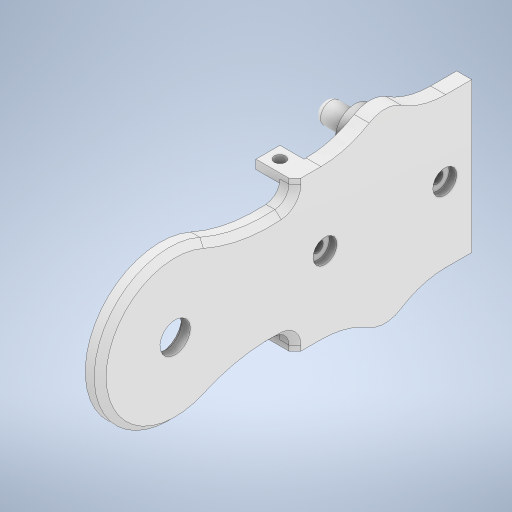
# Autodesk Inventor part: bldc_arm
Saved by Autodesk Inventor 2024.2 (Build 282272000, 272)
## iProperties
Created: 2024-03-15
Part Number: bldc_arm
Material: ABS Plastic
Document SubType Name: Modeling
Designer: jerem
Density: 1.06 g/cm^3
Appearance: Smooth - White
Mass: 32.0643 g
Surface Area: 145.548 cm^2
Volume: 30.2494 cm^3
Author: jerem
Autodesk Inventor part; units mm, degrees
ref_plane "YZ Plane" through (0, 0, 0) normal (1, 0, 0) x (0, 1, 0)
ref_plane "XZ Plane" through (0, 0, 0) normal (0, 1, 0) x (-1, 0, 0)
ref_plane "XY Plane" through (0, 0, 0) normal (0, 0, 1) x (1, 0, 0)
sketch "Sketch1" plane through (0, 0, 0) normal (1, 0, 0) x (0, 1, 0)
  line L0 (0, 0) -> (0, -10) construction
  line L1 (0, -10) -> (0, -50) construction
  circle A0 centre (0, -10) radius 1.905
  circle A1 centre (0, -50) radius 1.905
  line L2 (10, 0) -> (10, -59)
  line L3 (10, -59) -> (0, -59)
  line L4 (0, -59) -> (-10, -59)
  line L5 (-10, -59) -> (-10, 0)
  line L6 (0, 0) -> (10, 0)
  line L7 (0, 0) -> (-10, 0)
  line L8 (0, -50) -> (0, -59) construction
  circle A2 centre (0, 40) radius 25
  line L9 (10, 0) -> (10, 10)
  line L10 (10, 10) -> (-10, 10)
  line L11 (-10, 10) -> (-10, 0)
  arc A3 (22.8049, 29.7561) -> (10, -30) centre (155.8333, -30) ccw
  arc A4 (-10, -30) -> (-22.8049, 29.7561) centre (-155.8333, -30) ccw
  line L12 (0, -30) -> (21, -30) construction
  line L13 (0, -30) -> (-21, -30) construction
  circle A5 centre (21, -30) radius 3.5
  circle A6 centre (-21, -30) radius 3.5
  circle A7 centre (21, -30) radius 10
  circle A8 centre (-21, -30) radius 10
  circle A9 centre (21, -30) radius 6.5
  circle A10 centre (-21, -30) radius 6.5
  line L14 (-10, -59) -> (-25, -59)
  line L15 (10, -59) -> (25, -59)
  arc A11 (-28.9586, -23.9452) -> (-22.8049, 29.7561) centre (-71.0556, 8.082) ccw
  arc A12 (22.8049, 29.7561) -> (28.9586, -23.9452) centre (71.0556, 8.082) ccw
  line L16 (0, 0) -> (15, 0)
  line L17 (10, 0) -> (25, 0)
  line L18 (25, -59) -> (25, -50.3)
  arc A13 (29.3932, -35.4364) -> (25, -50.3) centre (52.3408, -50.3) ccw
  line L19 (25, 0) -> (25, -8.7)
  arc A14 (25, -8.7) -> (29.5297, -24.7804) centre (55.8075, -8.7) ccw
  line L20 (-10, 0) -> (-25, 0)
  line L21 (-25, -59) -> (-25, -50.3)
  arc A15 (-25, -50.3) -> (-29.3932, -35.4364) centre (-52.3408, -50.3) ccw
  line L22 (-25, 0) -> (-25, -8.7)
  arc A16 (-29.5297, -24.7804) -> (-25, -8.7) centre (-55.8075, -8.7) ccw
  circle A17 centre (0, -50) radius 4
  circle A18 centre (0, -10) radius 4
  circle A19 centre (0, 40) radius 7.235
  circle A20 centre (0, 40) radius 5.08
  point P0 (-10, -30)
  point P1 (10, -30)
  point P2 (23.8246, -39.5928)
  point P3 (10, -63.336)
  point P4 (-30.2308, -33.8462)
  point P5 (28.9586, -23.9452)
  point P6 (22.8049, 29.7561)
  point P7 (30.2308, -26.1538)
  point P8 (18.7815, 0)
  point P9 (-18.7815, 0)
  point P10 (-13.1191, 0)
  point P11 (-29.3932, -35.4364)
  dimension "d0" = 3.81
  dimension "d1" = 3.81
  dimension "d2" = 40
  dimension "d3" = 10
  dimension "d5" = 9
  dimension "d7" = 10
  dimension "d8" = 10
  dimension "d9" = 50
  dimension "d12" = 30
  dimension "d13" = 10
  dimension "d14" = 20
  dimension "d30" = 21
  dimension "d31" = 7
  dimension "d32" = 7
  dimension "d33" = 20
  dimension "d34" = 20
  dimension "d38" = 3
  dimension "d48" = 15
  dimension "d55" = 15
  dimension "d56" = 8.7
  dimension "d57" = 8.7
  dimension "d58" = 15
  dimension "d134" = 8
  dimension "d135" = 8
  dimension "d138" = 14.47
  dimension "d157" = 10.16
  constraints: 47 end point, 25 point on circle, 21 centre point, 14 symmetric about line, 11 coincident, 8 point on line, 8 tangent, 6 perpendicular, 5 horizontal, 5 vertical, 4 equal length, 1 midpoint, 5 other
  measures "d0" diameter of A0
  measures "d1" diameter of A1
  measures "d2" distance of L0.end L1.end
  measures "d3" distance of L0.start L0.end
  measures "d5" distance of L3.end L1.end
  measures "d7" distance from line of L12.start L5
  measures "d8" distance between parallel lines of L1 L2
  measures "d9" diameter of A2
  measures "d12" distance from line of A2.centre L10
  measures "d13" distance of L2.start L9.end
  measures "d14" vertical distance of L0.end A3.end
  measures "d30" distance of L12.start L12.end
  measures "d31" diameter of A5
  measures "d32" diameter of A6
  measures "d33" diameter of A7
  measures "d34" diameter of A8
  measures "d38" radial gap between concentric circles of A9 A5
  measures "d48" distance of L4.end L14.end
  measures "d55" distance of L2.start L17.end
  measures "d56" distance of L15.end L18.end
  measures "d57" distance of L17.end L19.end
  measures "d58" distance of L2.end L15.end
  measures "d134" diameter of A17
  measures "d135" diameter of A18
  measures "d138" diameter of A19
  measures "d157" diameter of A20
extrude "Extrusion1" add sketch "Sketch1" along normal blind 5 contours L16 A3 L2 | L2 L3 L4 L5 L7 L6 | L6 L7 L11 L10 L9 | L9 L10 L11 L20 A4 A2 A3 L16 | A3 L16 L17 A12 A7 A13 L18 L15 L2 | A3 A12 L17 L16 | L5 A4 L20 | A2 | L5 L14 L21 A15 A8 A11 L20 A4 | L20 A11 A4 | L17 L19 A14 A7 A12 | A11 A8 A16 L22 L20 | A7 | A8 | A5 | A6 | A9 | A10 | A17 | A18 | A19 | A20
fillet "Face Fillet1" radius 5 1 edges at (2.5, -18.7815, 0)
fillet "Face Fillet2" radius 5 1 edges at (2.5, 18.7815, 0)
extrude "Extrusion16" cut sketch "Sketch1" along normal up to surface (5 mm away) contours A20
extrude "Extrusion17" cut sketch "Sketch1" along normal blind 2 from surface at 0 contours A19 | A20
extrude "Extrusion11" cut sketch "Sketch1" against normal blind 2.5 from surface at 5 contours A17 | A18
extrude "Extrusion19" add sketch "Sketch1" against normal blind 15 contours A5 | A6
extrude "Extrusion20" add sketch "Sketch1" against normal blind 5 contours A9 | A10
fillet "Fillet4" radius 2 2 edges at (-15, 17.5, -30) (-15, -24.5, -30)
chamfer "Chamfer2" distance 2 angle 45 7 edges at (5, 0, 65) (5, -19.0046, 17.4944) (5, -19.8398, 1.3525) (5, -24.1298, 0) (5, 19.0046, 17.4944) (5, 19.8398, 1.3525) (5, 24.1298, 0)
sketch "Sketch15" plane through (0, 0, 0) normal (-1, 0, 0) x (0, 0, 1)
  line L0 (0, 25) -> (0, 23.2597) projected
  line L1 (0, 25) -> (-8, 25)
  line L2 (-8, 25) -> (-8, 22)
  line L3 (-8, 22) -> (0, 22)
  line L4 (0, 22) -> (0, 25)
  point P0 (0, 0)
  dimension "d175" = 8
  dimension "d176" = 3
  constraints: 8 end point, 2 parallel, 1 horizontal, 1 perpendicular
  measures "d175" distance of L3.end L2.end
  measures "d176" distance of L2.end L1.end
extrude "Extrusion21" add sketch "Sketch15" along normal blind 8
sketch "Sketch16" plane through (0, 25, -8.7) normal (0, 1, 0) x (1, 0, 0)
  circle A0 centre (-4, -4.7) radius 1.905
  line L0 (-8, -8.7) -> (-8, -0.7) projected
  line L1 (-8, -8.7) -> (3, -8.7) projected
  point P0 (0, -8.7)
  dimension "d179" = 3.81
  dimension "d180" = 4
  dimension "d181" = 4
  constraints: 1 centre point
  measures "d179" diameter of A0
  measures "d180" distance from line of L0 A0.centre
  measures "d181" distance from line of L1 A0.centre
extrude "Extrusion22" cut sketch "Sketch16" against normal up to surface (3 mm away)
mirror "Mirror2" about plane through (0, 0, 0) normal (0, 1, 0) of "Extrusion22", "Extrusion21"
equation "\"d0\" = M4_HOLE_D"
equation "\"d1\" = d0"
equation "\"d14\" = 0.5 * d2"
equation "\"d32\" = d31"
equation "\"d34\" = d33"
equation "\"M4_HOLE_D\" = 3.81"
equation "\"M3_HOLE_D\" = 2.54"
equation "\"d88\" = 3"
body "Solid1"
